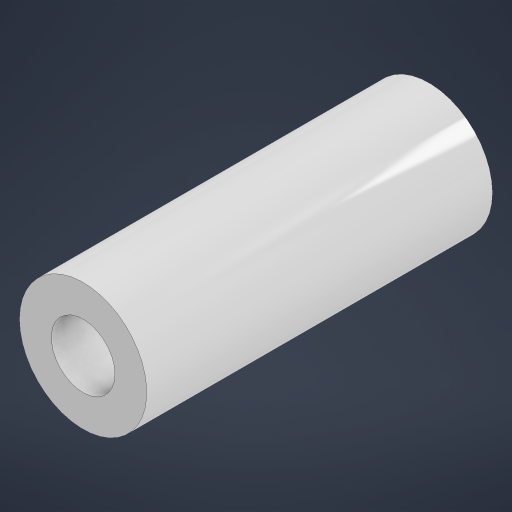
# Autodesk Inventor part: spacer_2020_node
Saved by Autodesk Inventor 2024 (Build 280153000, 153)
## iProperties
Created: 2026-03-28
Part Number: spacer_2020_node
Material: PET Plastic
Document SubType Name: Modeling
Designer: schar
Density: 1.541 g/cm^3
Appearance: Polycarbonate - Clear
Author: schar
Autodesk Inventor part; units mm, degrees
ref_plane "YZ Plane" through (0, 0, 0) normal (1, 0, 0) x (0, 1, 0)
ref_plane "XZ Plane" through (0, 0, 0) normal (0, 1, 0) x (-1, 0, 0)
sketch "Sketch1" plane through (0, 0, 0) normal (0, 0, 1) x (1, 0, 0)
  circle A0 centre (-2.1639, -8.8533) radius 2.5 projected
  circle A1 centre (-2.1639, -8.8533) radius 2.5
  circle A2 centre (-2.164, -8.8536) radius 5 projected
  circle A3 centre (-2.164, -8.8536) radius 5
  point P0 (0, 0)
  constraints: 2 centre point, 2 coincident, 2 concentric
ref_plane "Work Plane1" through (-131.0962, -66.9734, 27.172) normal (0, 0, -1) x (-0.5, 0.866, 0)
extrude "Extrusion1" add sketch "Sketch1" along normal up to surface (27.172 mm away)
body "Solid1"
